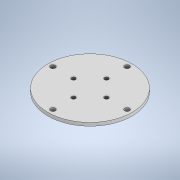
# Autodesk Inventor part: 판
Saved by Autodesk Inventor 2020 (Build 240168000, 168)
## iProperties
Created: 2020-05-01
Part Number: 판
Material: Generic
Document SubType Name: Modeling
Designer: introbot
Density: 1 g/cm^3
Appearance: Default
Author: introbot
Autodesk Inventor part; units mm, degrees
ref_plane "YZ Plane" through (0, 0, 0) normal (1, 0, 0) x (0, 1, 0)
ref_plane "XZ Plane" through (0, 0, 0) normal (0, 1, 0) x (-1, 0, 0)
ref_plane "XY Plane" through (0, 0, 0) normal (0, 0, 1) x (1, 0, 0)
sketch "Sketch1" plane through (0, 0, 0) normal (0, 1, 0) x (-1, 0, 0)
  point P0 (0, 0)
sketch "Sketch2" plane through (0, 0, 0) normal (0, 1, 0) x (-1, 0, 0)
  circle A0 centre (0, 0) radius 25.5
  dimension "d0" = 51
  constraints: 1 centre point, 1 coincident
  measures "d0" diameter of A0
extrude "Extrusion1" add sketch "Sketch2" along normal blind 2
sketch "Sketch3" plane through (0, 2, 0) normal (0, 1, 0) x (1, 0, 0)
  circle A0 centre (0, 0) radius 22.5
  line L0 (-35.7, 0) -> (35.7, 0) projected
  line L1 (0, 35.7) -> (0, -35.7) projected
  point P0 (-22.5, 0)
  point P1 (0, -22.5)
  point P2 (22.5, 0)
  point P3 (0, 22.5)
  dimension "d3" = 45
  constraints: 4 point on circle, 4 point on line, 1 centre point, 1 coincident
  measures "d3" diameter of A0
hole "Hole1" at (-22.5, 2, 0) at (0, 2, 22.5) at (22.5, 2, 0) at (0, 2, -22.5) direction (0, -1, 0) diameter 3 end through all
sketch "Sketch4" plane through (0, 2, 0) normal (0, 1, 0) x (1, 0, 0)
  circle A0 centre (0, 0) radius 10
  point P0 (0, -10)
  point P1 (10, 0)
  point P2 (0, 10)
  point P3 (-10, 0)
  dimension "d11" = 20
  constraints: 4 point on circle, 1 centre point, 1 coincident
  measures "d11" diameter of A0
hole "Hole2" at (-10, 2, 0) at (0, 2, 10) at (10, 2, 0) at (0, 2, -10) direction (0, -1, 0) diameter 2.459 end through all thread size "M3x0.5" class "6H" standard "ANSI Metric M Profile"
body "Solid1"
